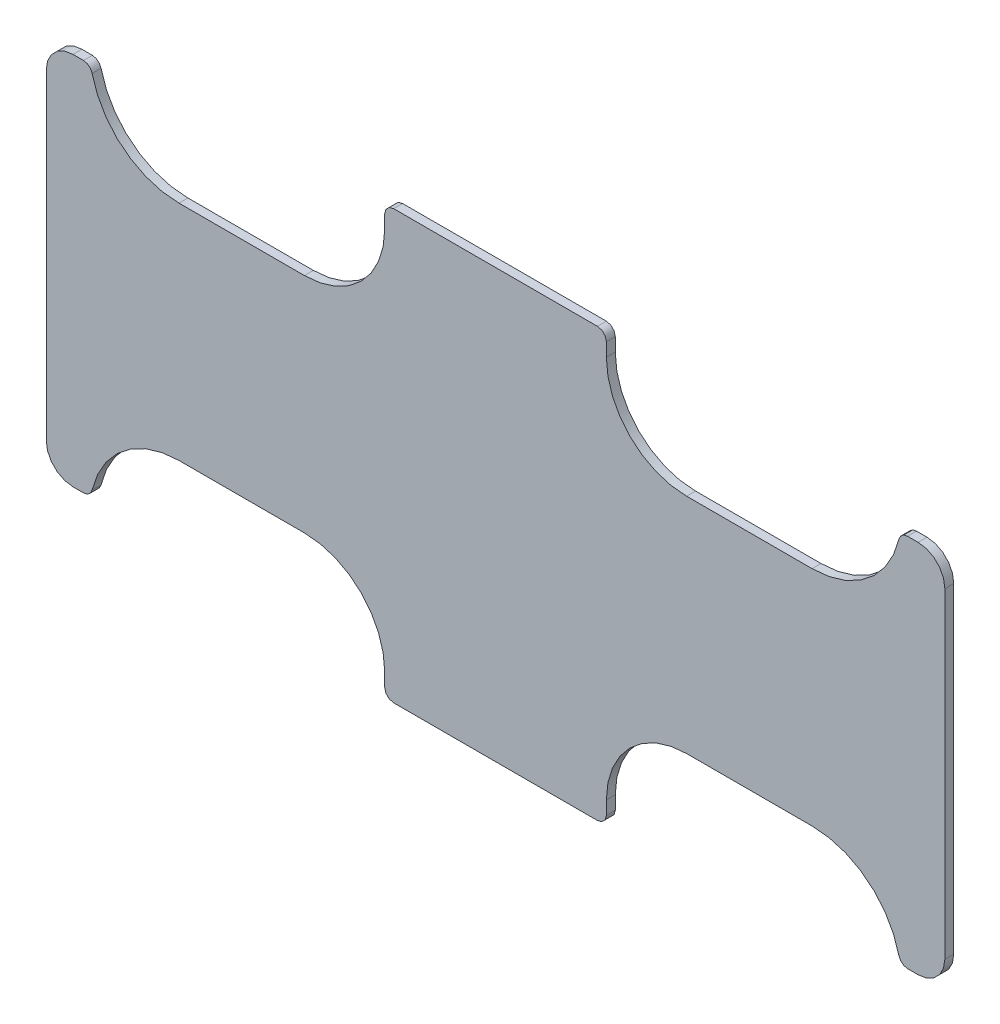
# Autodesk Inventor part: my_base
Saved by Autodesk Inventor 2020.2 (Build 242310000, 310)
## iProperties
Created: 2021-06-23
Part Number: my_base
Material: Generic
Document SubType Name: Modeling
Designer: Tarsoly
Density: 1 g/cm^3
Appearance: Default
Author: Tarsoly
Autodesk Inventor part; units mm, degrees
ref_plane "YZ Plane" through (0, 0, 0) normal (1, 0, 0) x (0, 1, 0)
ref_plane "XZ Plane" through (0, 0, 0) normal (0, 1, 0) x (-1, 0, 0)
ref_plane "XY Plane" through (0, 0, 0) normal (0, 0, 1) x (1, 0, 0)
sketch "Sketch1" plane through (0, 0, 0) normal (0, 0, 1) x (1, 0, 0)
  line L0 (323.3438, -62.5) -> (393.7095, -62.5) projected
  arc A0 (323.3438, -62.5) -> (278.3438, -107.5) centre (323.3438, -107.5) ccw projected
  line L1 (278.3438, -115) -> (278.3438, -107.5) projected
  arc A1 (273.3438, -120) -> (278.3438, -115) centre (273.3438, -115) ccw projected
  line L2 (149.8438, -120) -> (273.3438, -120) projected
  arc A2 (442.4011, -101.1364) -> (393.7095, -62.5) centre (393.7095, -112.5) ccw projected
  arc A3 (442.4011, -101.1364) -> (447.2702, -105) centre (447.2702, -100) ccw projected
  line L3 (453.1438, -105) -> (447.2702, -105) projected
  arc A4 (453.1438, -105) -> (468.1438, -90) centre (453.1438, -90) ccw projected
  line L4 (468.1438, 90) -> (468.1438, -90) projected
  arc A5 (468.1438, 90) -> (453.1438, 105) centre (453.1438, 90) ccw projected
  line L5 (447.2702, 105) -> (453.1438, 105) projected
  arc A6 (447.2702, 105) -> (442.4011, 101.1364) centre (447.2702, 100) ccw projected
  arc A7 (393.7095, 62.5) -> (442.4011, 101.1364) centre (393.7095, 112.5) ccw projected
  line L6 (393.7095, 62.5) -> (323.3438, 62.5) projected
  arc A8 (278.3438, 107.5) -> (323.3438, 62.5) centre (323.3438, 107.5) ccw projected
  line L7 (278.3438, 107.5) -> (278.3438, 115) projected
  arc A9 (278.3438, 115) -> (273.3438, 120) centre (273.3438, 115) ccw projected
  line L8 (273.3438, 120) -> (149.8438, 120) projected
  arc A10 (149.8438, 120) -> (144.8438, 115) centre (149.8438, 115) ccw projected
  line L9 (144.8438, 115) -> (144.8438, 107.5) projected
  arc A11 (124.8438, 87.5) -> (144.8438, 107.5) centre (124.8438, 107.5) ccw projected
  line L10 (106.6438, 87.5) -> (124.8438, 87.5) projected
  arc A12 (106.6438, 87.5) -> (101.6438, 82.5) centre (106.6438, 82.5) ccw projected
  line L11 (101.6438, 82.5) -> (101.6438, 63.25) projected
  arc A13 (96.6438, 58.25) -> (101.6438, 63.25) centre (96.6438, 63.25) ccw projected
  line L12 (91.6516, 58.25) -> (96.6438, 58.25) projected
  arc A14 (91.6516, 58.25) -> (85.6702, 54.8864) centre (91.6516, 51.25) ccw projected
  arc A15 (62.0674, 54.8864) -> (85.6702, 54.8864) centre (73.8688, 62.0613) ccw projected
  arc A16 (62.0674, 54.8864) -> (56.0861, 58.25) centre (56.0861, 51.25) ccw projected
  line L13 (56.0861, 58.25) -> (45.5938, 58.25) projected
  arc A17 (40.5938, 63.25) -> (45.5938, 58.25) centre (45.5938, 63.25) ccw projected
  line L14 (40.5938, 82.5) -> (40.5938, 63.25) projected
  arc A18 (40.5938, 82.5) -> (35.5938, 87.5) centre (35.5938, 82.5) ccw projected
  line L15 (10.1649, 87.5) -> (35.5938, 87.5) projected
  arc A19 (10.1649, 87.5) -> (5.2408, 83.3682) centre (10.1649, 82.5) ccw projected
  line L16 (-2.4062, 40) -> (5.2408, 83.3682) projected
  line L17 (-2.4062, -40) -> (-2.4062, 40) projected
  line L18 (-2.4062, -40) -> (5.2408, -83.3682) projected
  arc A20 (5.2408, -83.3682) -> (10.1649, -87.5) centre (10.1649, -82.5) ccw projected
  line L19 (35.5938, -87.5) -> (10.1649, -87.5) projected
  arc A21 (35.5938, -87.5) -> (40.5938, -82.5) centre (35.5938, -82.5) ccw projected
  line L20 (40.5938, -63.25) -> (40.5938, -82.5) projected
  arc A22 (45.5938, -58.25) -> (40.5938, -63.25) centre (45.5938, -63.25) ccw projected
  line L21 (56.0861, -58.25) -> (45.5938, -58.25) projected
  arc A23 (56.0861, -58.25) -> (62.0674, -54.8864) centre (56.0861, -51.25) ccw projected
  arc A24 (85.6702, -54.8864) -> (62.0674, -54.8864) centre (73.8688, -62.0613) ccw projected
  arc A25 (85.6702, -54.8864) -> (91.6516, -58.25) centre (91.6516, -51.25) ccw projected
  line L22 (91.6516, -58.25) -> (96.6438, -58.25) projected
  arc A26 (101.6438, -63.25) -> (96.6438, -58.25) centre (96.6438, -63.25) ccw projected
  line L23 (101.6438, -82.5) -> (101.6438, -63.25) projected
  arc A27 (101.6438, -82.5) -> (106.6438, -87.5) centre (106.6438, -82.5) ccw projected
  line L24 (106.6438, -87.5) -> (124.8438, -87.5) projected
  arc A28 (144.8438, -107.5) -> (124.8438, -87.5) centre (124.8438, -107.5) ccw projected
  line L25 (144.8438, -115) -> (144.8438, -107.5) projected
  arc A29 (144.8438, -115) -> (149.8438, -120) centre (149.8438, -115) ccw projected
  line L26 (216.1977, -168) -> (216.1977, 168)
  line L27 (109.0517, -62.5) -> (38.686, -62.5)
  arc A30 (154.0517, -107.5) -> (109.0517, -62.5) centre (109.0517, -107.5) ccw
  line L28 (154.0517, -115) -> (154.0517, -107.5)
  arc A31 (154.0517, -115) -> (159.0517, -120) centre (159.0517, -115) ccw
  line L29 (282.5517, -120) -> (159.0517, -120)
  arc A32 (38.686, -62.5) -> (-10.0056, -101.1364) centre (38.686, -112.5) ccw
  arc A33 (-14.8747, -105) -> (-10.0056, -101.1364) centre (-14.8747, -100) ccw
  line L30 (-20.7483, -105) -> (-14.8747, -105)
  arc A34 (-35.7483, -90) -> (-20.7483, -105) centre (-20.7483, -90) ccw
  line L31 (-35.7483, 90) -> (-35.7483, -90)
  arc A35 (-20.7483, 105) -> (-35.7483, 90) centre (-20.7483, 90) ccw
  line L32 (-14.8747, 105) -> (-20.7483, 105)
  arc A36 (-10.0056, 101.1364) -> (-14.8747, 105) centre (-14.8747, 100) ccw
  arc A37 (-10.0056, 101.1364) -> (38.686, 62.5) centre (38.686, 112.5) ccw
  line L33 (38.686, 62.5) -> (109.0517, 62.5)
  arc A38 (109.0517, 62.5) -> (154.0517, 107.5) centre (109.0517, 107.5) ccw
  line L34 (154.0517, 107.5) -> (154.0517, 115)
  arc A39 (159.0517, 120) -> (154.0517, 115) centre (159.0517, 115) ccw
  line L35 (159.0517, 120) -> (282.5517, 120)
  arc A40 (287.5517, 115) -> (282.5517, 120) centre (282.5517, 115) ccw
  line L36 (287.5517, 115) -> (287.5517, 107.5)
  arc A41 (287.5517, 107.5) -> (307.5517, 87.5) centre (307.5517, 107.5) ccw
  line L37 (325.7517, 87.5) -> (307.5517, 87.5)
  arc A42 (330.7517, 82.5) -> (325.7517, 87.5) centre (325.7517, 82.5) ccw
  line L38 (330.7517, 82.5) -> (330.7517, 63.25)
  arc A43 (330.7517, 63.25) -> (335.7517, 58.25) centre (335.7517, 63.25) ccw
  line L39 (340.7439, 58.25) -> (335.7517, 58.25)
  arc A44 (346.7253, 54.8864) -> (340.7439, 58.25) centre (340.7439, 51.25) ccw
  arc A45 (346.7253, 54.8864) -> (370.3281, 54.8864) centre (358.5267, 62.0613) ccw
  arc A46 (376.3094, 58.25) -> (370.3281, 54.8864) centre (376.3094, 51.25) ccw
  line L40 (376.3094, 58.25) -> (386.8017, 58.25)
  arc A47 (386.8017, 58.25) -> (391.8017, 63.25) centre (386.8017, 63.25) ccw
  line L41 (391.8017, 82.5) -> (391.8017, 63.25)
  arc A48 (396.8017, 87.5) -> (391.8017, 82.5) centre (396.8017, 82.5) ccw
  line L42 (422.2306, 87.5) -> (396.8017, 87.5)
  arc A49 (427.1547, 83.3682) -> (422.2306, 87.5) centre (422.2306, 82.5) ccw
  line L43 (434.8017, 40) -> (427.1547, 83.3682)
  line L44 (434.8017, -40) -> (434.8017, 40)
  line L45 (434.8017, -40) -> (427.1547, -83.3682)
  arc A50 (422.2306, -87.5) -> (427.1547, -83.3682) centre (422.2306, -82.5) ccw
  line L46 (396.8017, -87.5) -> (422.2306, -87.5)
  arc A51 (391.8017, -82.5) -> (396.8017, -87.5) centre (396.8017, -82.5) ccw
  line L47 (391.8017, -63.25) -> (391.8017, -82.5)
  arc A52 (391.8017, -63.25) -> (386.8017, -58.25) centre (386.8017, -63.25) ccw
  line L48 (376.3094, -58.25) -> (386.8017, -58.25)
  arc A53 (370.3281, -54.8864) -> (376.3094, -58.25) centre (376.3094, -51.25) ccw
  arc A54 (370.3281, -54.8864) -> (346.7253, -54.8864) centre (358.5267, -62.0613) ccw
  arc A55 (340.7439, -58.25) -> (346.7253, -54.8864) centre (340.7439, -51.25) ccw
  line L49 (340.7439, -58.25) -> (335.7517, -58.25)
  arc A56 (335.7517, -58.25) -> (330.7517, -63.25) centre (335.7517, -63.25) ccw
  line L50 (330.7517, -82.5) -> (330.7517, -63.25)
  arc A57 (325.7517, -87.5) -> (330.7517, -82.5) centre (325.7517, -82.5) ccw
  line L51 (325.7517, -87.5) -> (307.5517, -87.5)
  arc A58 (307.5517, -87.5) -> (287.5517, -107.5) centre (307.5517, -107.5) ccw
  line L52 (287.5517, -115) -> (287.5517, -107.5)
  arc A59 (282.5517, -120) -> (287.5517, -115) centre (282.5517, -115) ccw
  point P0 (0, 0)
  point P1 (432.3955, 0)
  constraints: 87 symmetric about line, 60 point on circle, 54 end point, 30 centre point, 1 vertical, 32 other
extrude "Extrusion1" add sketch "Sketch1" against normal blind 5 contours A0 L1 A1 L2 L26 L8 A9 L7 A8 L6 A43 L39 A44 A45 A46 L40 A47 A7 L43 L44 L45 A2 L0 A52 L48 A53 A54 A55 L49 A56 | A56 L49 A55 A54 A53 L48 A52 L0 | L45 L44 L43 A7 A6 L5 A5 L4 A4 L3 A3 A2 | L2 A31 L28 A30 L27 A26 L22 A25 A24 A23 L21 A22 A32 L18 L17 L16 A37 L33 A17 L13 A16 A15 A14 L12 A13 A38 L34 A39 L8 L26 | A47 L40 A46 A45 A44 L39 A43 L6 | L27 A22 L21 A23 A24 A25 L22 A26 | A13 L12 A14 A15 A16 L13 A17 L33 | A32 A33 L30 A34 L31 A35 L32 A36 A37 L16 L17 L18
body "Solid1"
